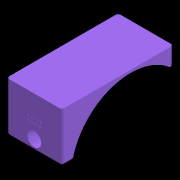
# Autodesk Inventor part: strut_hole
Saved by Autodesk Inventor 2020.2 (Build 242310000, 310)
## iProperties
Created: 2020-04-29
Part Number: strut_hole
Material: PC/ABS Plastic
Document SubType Name: Modeling
Designer: agmlego
Mass: 206.183 g
Surface Area: 707.007 cm^2
Volume: 577.101 cm^3
Density: 0.357273 g/cm^3
Appearance: Violet
Author: agmlego
Autodesk Inventor part; units mm, degrees
ref_plane "YZ Plane" through (0, 0, 0) normal (1, 0, 0) x (0, 1, 0)
ref_plane "XZ Plane" through (0, 0, 0) normal (0, 1, 0) x (-1, 0, 0)
ref_plane "XY Plane" through (0, 0, 0) normal (0, 0, 1) x (1, 0, 0)
sketch "Sketch1" plane through (0, 0, 0) normal (1, 0, 0) x (0, 1, 0)
  arc A0 (76.4375, -78.4587) -> (23.4861, 106.99) centre (0, 0) ccw
  line L0 (114.5375, 126.6449) -> (76.4375, 126.6449)
  line L1 (76.4375, -78.4587) -> (114.5375, -78.4587)
  line L2 (114.5375, -78.4587) -> (114.5375, 126.6449)
  line L3 (114.5375, 0) -> (109.5375, 0) construction
  line L4 (55.1307, 126.6449) -> (28.4861, 126.6449) construction
  line L5 (28.4861, 126.6449) -> (28.4861, 75.8449) construction
  line L6 (28.4861, 75.8449) -> (55.1307, 75.8449) construction
  line L7 (55.1307, 75.8449) -> (55.1307, 126.6449) construction
  line L8 (41.8084, 75.8449) -> (41.8084, 126.6449) construction
  line L9 (76.4375, 126.6449) -> (23.4861, 126.6449)
  line L10 (23.4861, 126.6449) -> (23.4861, 106.99)
  point P0 (41.8084, 101.2449)
  dimension "d0" = 219.075
  dimension "d1" = 38.1
  dimension "d3" = 5
  dimension "d4" = 26.6446
  dimension "d5" = 41.8084
  dimension "d6" = 25.4
  dimension "d7" = 5
  constraints: 22 end point, 4 horizontal, 4 parallel, 4 point on circle, 3 midpoint, 2 perpendicular, 2 point on line, 1 centre point, 1 coincident, 1 collinear, 1 vertical
  measures "d0" diameter of A0
  measures "d1" distance of L0.start L0.end
  measures "d3" distance of L3.start L3.end
  measures "d4" distance of L4.start L4.end
  measures "d5" distance from line of point (0, 0) L8
  measures "d6" distance from line of point (41.808, 101.245) L4
  measures "d7" distance between parallel lines of L5 L10
extrude "Extrusion1" add sketch "Sketch1" along normal blind 101.6
sketch "Sketch3" plane through (0, 23.4861, 126.6449) normal (0, 0, 1) x (1, 0, 0)
  line L0 (0, 18.3223) -> (101.6, 18.3223) construction
  line L1 (101.6, 86.0514) -> (101.6, 0) construction
  point P0 (0, -23.4861)
  point P1 (50.8, 18.3223)
  point P2 (101.6, 52.9514)
  point P3 (50.8, 18.3223)
  dimension "d10" = 41.8084
  constraints: 2 end point, 1 coincident, 1 horizontal, 1 midpoint, 1 point on line
  measures "d10" distance from line of point (0, -23.486) L0
hole "Hole1" at (50.8, 41.8084, 126.6449) direction (0, 0, -1) diameter 25.4 end through all
fillet "Fillet1" radius 5 9 edges at (50.8, 76.4375, -78.4587) (0, 95.4875, -78.4587) (101.6, 95.4875, -78.4587) (0, 69.0118, 126.6449) (50.8, 23.4861, 106.99) (0, 23.4861, 116.8174) (50.8, 23.4861, 126.6449) (101.6, 69.0118, 126.6449) (101.6, 23.4861, 116.8174)
sketch "Sketch4" plane through (5, 28.4861, 126.6449) normal (0, 0, 1) x (1, 0, 0)
  line L0 (32.0406, 47.3735) -> (60.3413, 47.3735) construction
  line L1 (60.3413, 47.3735) -> (60.3413, 37.5666) construction
  line L2 (60.3413, 37.5666) -> (32.0406, 37.5666) construction
  line L3 (32.0406, 37.5666) -> (32.0406, 47.3735) construction
  spline S0 degree 2 poles (35.6936, 46.8807) (35.5562, 46.9611) (35.3046, 47.0363) (35.1516, 47.0363) knots 0 0 0 1 2 2 2
  spline S1 degree 2 poles (35.1516, 47.0363) (35.0426, 47.0363) (34.8352, 46.9922) (34.677, 46.8937) (34.5784, 46.7355) (34.5784, 46.6214) knots 0 0 0 1 2 3 4 4 4
  spline S2 degree 2 poles (34.5784, 46.6214) (34.5784, 46.5098) (34.6977, 46.3439) (34.8922, 46.2142) (35.1438, 46.1027) (35.4057, 45.9808) (35.6573, 45.8355) (35.8518, 45.6358) (35.9711, 45.3713) (35.9711, 45.1897) knots 0 0 0 1 2 3 4 5 6 7 8 8 8
  spline S3 degree 2 poles (35.9711, 45.1897) (35.9711, 45.0419) (35.8907, 44.7903) (35.7481, 44.5906) (35.551, 44.4402) (35.3176, 44.339) (35.0608, 44.2898) (34.9259, 44.2898) knots 0 0 0 1 2 3 4 5 6 6 6
  spline S4 degree 2 poles (34.9259, 44.2898) (34.4565, 44.2976) (34.109, 44.5128) knots 0 0 0 1 1 1
  line L4 (34.109, 44.5128) -> (34.2931, 44.8137)
  spline S5 degree 2 poles (34.2931, 44.8137) (34.332, 44.7877) (34.4643, 44.7229) (34.6251, 44.6606) (34.804, 44.6217) (34.8974, 44.6217) knots 0 0 0 1 2 3 4 4 4
  spline S6 degree 2 poles (34.8974, 44.6217) (35.0219, 44.6217) (35.2605, 44.684) (35.4472, 44.8137) (35.5613, 45.016) (35.5613, 45.1534) knots 0 0 0 1 2 3 4 4 4
  spline S7 degree 2 poles (35.5613, 45.1534) (35.5613, 45.2831) (35.442, 45.4776) (35.2475, 45.6332) (34.996, 45.7577) (34.734, 45.8822) (34.4824, 46.0171) (34.2879, 46.1908) (34.1686, 46.4139) (34.1686, 46.5643) knots 0 0 0 1 2 3 4 5 6 7 8 8 8
  spline S8 degree 2 poles (34.1686, 46.5643) (34.1686, 46.7588) (34.3294, 47.0571) (34.5914, 47.262) (34.9259, 47.3683) (35.0971, 47.3683) knots 0 0 0 1 2 3 4 4 4
  spline S9 degree 2 poles (35.0971, 47.3683) (35.525, 47.3683) (35.8881, 47.1271) knots 0 0 0 1 1 1
  line L5 (35.8881, 47.1271) -> (35.6936, 46.8807)
  line L6 (37.146, 44.3235) -> (37.146, 47.013)
  line L7 (37.146, 47.013) -> (36.3135, 47.013)
  line L8 (36.3135, 47.013) -> (36.3135, 47.3346)
  line L9 (36.3135, 47.3346) -> (38.3909, 47.3346)
  line L10 (38.3909, 47.3346) -> (38.3909, 47.013)
  line L11 (38.3909, 47.013) -> (37.5687, 47.013)
  line L12 (37.5687, 47.013) -> (37.5687, 44.3235)
  line L13 (37.5687, 44.3235) -> (37.146, 44.3235)
  line L14 (39.3661, 45.5554) -> (39.3661, 44.3235)
  line L15 (39.3661, 44.3235) -> (38.9433, 44.3235)
  line L16 (38.9433, 44.3235) -> (38.9433, 46.9118)
  line L17 (38.9433, 46.9118) -> (38.8733, 47.3138)
  spline S10 degree 2 poles (38.8733, 47.3138) (38.9381, 47.3216) (39.1249, 47.3372) (39.3298, 47.3501) (39.5321, 47.3579) (39.6202, 47.3579) knots 0 0 0 1 2 3 4 4 4
  spline S11 degree 2 poles (39.6202, 47.3579) (39.8718, 47.3579) (40.2894, 47.2516) (40.5876, 47.0441) (40.751, 46.7329) (40.751, 46.528) knots 0 0 0 1 2 3 4 4 4
  spline S12 degree 2 poles (40.751, 46.528) (40.751, 46.3179) (40.6213, 45.9963) (40.3827, 45.7707) (40.0559, 45.628) (39.8614, 45.5943) knots 0 0 0 1 2 3 4 4 4
  line L18 (39.8614, 45.5943) -> (40.1467, 45.5139)
  line L19 (40.1467, 45.5139) -> (41.0363, 44.3235)
  line L20 (41.0363, 44.3235) -> (40.5876, 44.3235)
  line L21 (40.5876, 44.3235) -> (39.7006, 45.5165)
  spline S13 degree 2 poles (39.7006, 45.5165) (39.6773, 45.545) (39.6228, 45.5554) (39.6073, 45.5554) knots 0 0 0 1 2 2 2
  line L22 (39.6073, 45.5554) -> (39.3661, 45.5554)
  line L23 (39.3661, 46.624) -> (39.3661, 45.8589)
  line L24 (39.3661, 45.8589) -> (39.6617, 45.8589)
  spline S14 degree 2 poles (39.6617, 45.8589) (39.8459, 45.8589) (40.113, 45.96) (40.2894, 46.1364) (40.3775, 46.3672) (40.3775, 46.4969) knots 0 0 0 1 2 3 4 4 4
  spline S15 degree 2 poles (40.3775, 46.4969) (40.3775, 46.668) (40.2505, 46.8937) (40.0456, 47.0285) (39.794, 47.083) (39.6695, 47.083) knots 0 0 0 1 2 3 4 4 4
  spline S16 degree 2 poles (39.6695, 47.083) (39.628, 47.083) (39.5372, 47.0804) (39.4439, 47.0778) (39.3583, 47.0649) (39.3272, 47.0597) knots 0 0 0 1 2 3 4 4 4
  line L25 (39.3272, 47.0597) -> (39.3661, 46.624)
  line L26 (43.6221, 47.3346) -> (43.6221, 45.3739)
  spline S17 degree 2 poles (43.6221, 45.3739) (43.6221, 45.1015) (43.4561, 44.6944) (43.1708, 44.4246) (42.7766, 44.2898) (42.5457, 44.2898) knots 0 0 0 1 2 3 4 4 4
  spline S18 degree 2 poles (42.5457, 44.2898) (42.302, 44.2898) (41.9233, 44.4609) (41.6665, 44.7722) (41.5317, 45.2079) (41.5317, 45.4724) knots 0 0 0 1 2 3 4 4 4
  line L27 (41.5317, 45.4724) -> (41.5317, 46.9118)
  line L28 (41.5317, 46.9118) -> (41.472, 47.3346)
  line L29 (41.472, 47.3346) -> (41.944, 47.3735)
  line L30 (41.944, 47.3735) -> (41.944, 45.4361)
  spline S19 degree 2 poles (41.944, 45.4361) (41.944, 45.2468) (42.0452, 44.9459) (42.2164, 44.741) (42.4394, 44.6321) (42.5665, 44.6321) knots 0 0 0 1 2 3 4 4 4
  spline S20 degree 2 poles (42.5665, 44.6321) (42.7143, 44.6321) (42.9529, 44.7203) (43.1189, 44.8967) (43.2097, 45.1586) (43.2097, 45.3376) knots 0 0 0 1 2 3 4 4 4
  line L31 (43.2097, 45.3376) -> (43.2097, 47.3346)
  line L32 (43.2097, 47.3346) -> (43.6221, 47.3346)
  line L33 (44.9759, 44.3235) -> (44.9759, 47.013)
  line L34 (44.9759, 47.013) -> (44.1434, 47.013)
  line L35 (44.1434, 47.013) -> (44.1434, 47.3346)
  line L36 (44.1434, 47.3346) -> (46.2208, 47.3346)
  line L37 (46.2208, 47.3346) -> (46.2208, 47.013)
  line L38 (46.2208, 47.013) -> (45.3986, 47.013)
  line L39 (45.3986, 47.013) -> (45.3986, 44.3235)
  line L40 (45.3986, 44.3235) -> (44.9759, 44.3235)
  line L41 (49.8362, 44.3235) -> (49.8362, 45.7785)
  line L42 (49.8362, 45.7785) -> (48.5705, 45.7785)
  line L43 (48.5705, 45.7785) -> (48.5705, 44.3235)
  line L44 (48.5705, 44.3235) -> (48.1582, 44.3235)
  line L45 (48.1582, 44.3235) -> (48.1582, 46.9118)
  line L46 (48.1582, 46.9118) -> (48.1011, 47.3346)
  line L47 (48.1011, 47.3346) -> (48.5705, 47.3735)
  line L48 (48.5705, 47.3735) -> (48.5705, 46.1001)
  line L49 (48.5705, 46.1001) -> (49.8362, 46.1001)
  line L50 (49.8362, 46.1001) -> (49.8362, 47.3372)
  line L51 (49.8362, 47.3372) -> (50.2486, 47.3735)
  line L52 (50.2486, 47.3735) -> (50.2486, 44.3235)
  line L53 (50.2486, 44.3235) -> (49.8362, 44.3235)
  spline S21 degree 2 poles (52.2145, 44.2898) (51.898, 44.2898) (51.3949, 44.5232) (51.0448, 44.933) (50.858, 45.4984) (50.858, 45.8303) knots 0 0 0 1 2 3 4 4 4
  spline S22 degree 2 poles (50.858, 45.8303) (50.858, 46.1597) (51.0396, 46.7251) (51.3845, 47.1349) (51.8903, 47.3683) (52.2145, 47.3683) knots 0 0 0 1 2 3 4 4 4
  spline S23 degree 2 poles (52.2145, 47.3683) (52.5283, 47.3683) (53.034, 47.1349) (53.3841, 46.7251) (53.5709, 46.1597) (53.5709, 45.8303) knots 0 0 0 1 2 3 4 4 4
  spline S24 degree 2 poles (53.5709, 45.8303) (53.5709, 45.4984) (53.3893, 44.933) (53.0444, 44.5232) (52.5386, 44.2898) (52.2145, 44.2898) knots 0 0 0 1 2 3 4 4 4
  spline S25 degree 2 poles (53.1533, 45.7681) (53.1533, 45.9263) (53.1092, 46.2375) (53.0133, 46.5176) (52.8602, 46.7562) (52.6502, 46.9274) (52.3753, 47.026) (52.2015, 47.026) knots 0 0 0 1 2 3 4 5 6 6 6
  spline S26 degree 2 poles (52.2015, 47.026) (51.9551, 47.026) (51.605, 46.8366) (51.3793, 46.5176) (51.2756, 46.113) (51.2756, 45.9004) knots 0 0 0 1 2 3 4 4 4
  spline S27 degree 2 poles (51.2756, 45.9004) (51.2756, 45.737) (51.3223, 45.4231) (51.4182, 45.1404) (51.5687, 44.9018) (51.7787, 44.7307) (52.0537, 44.6321) (52.2274, 44.6321) knots 0 0 0 1 2 3 4 5 6 6 6
  spline S28 degree 2 poles (52.2274, 44.6321) (52.3882, 44.6321) (52.6528, 44.7229) (52.8602, 44.8785) (53.0081, 45.0964) (53.1066, 45.3453) (53.1533, 45.6254) (53.1533, 45.7681) knots 0 0 0 1 2 3 4 5 6 6 6
  line L54 (54.6031, 44.6451) -> (55.9076, 44.6451)
  line L55 (55.9076, 44.6451) -> (55.8687, 44.3235)
  line L56 (55.8687, 44.3235) -> (54.1622, 44.3235)
  line L57 (54.1622, 44.3235) -> (54.2011, 44.7255)
  line L58 (54.2011, 44.7255) -> (54.2011, 46.9118)
  line L59 (54.2011, 46.9118) -> (54.1415, 47.3346)
  line L60 (54.1415, 47.3346) -> (54.6238, 47.3735)
  line L61 (54.6238, 47.3735) -> (54.6238, 45.0056)
  line L62 (54.6238, 45.0056) -> (54.6031, 44.6451)
  line L63 (58.1251, 44.6451) -> (58.0862, 44.3235)
  line L64 (58.0862, 44.3235) -> (56.3771, 44.3235)
  line L65 (56.3771, 44.3235) -> (56.4082, 44.7255)
  line L66 (56.4082, 44.7255) -> (56.4082, 46.9118)
  line L67 (56.4082, 46.9118) -> (56.3486, 47.3346)
  line L68 (56.3486, 47.3346) -> (58.0551, 47.3346)
  line L69 (58.0551, 47.3346) -> (58.0551, 47.013)
  line L70 (58.0551, 47.013) -> (56.7895, 47.013)
  line L71 (56.7895, 47.013) -> (56.8309, 46.6317)
  line L72 (56.8309, 46.6317) -> (56.8309, 46.1001)
  line L73 (56.8309, 46.1001) -> (57.915, 46.1001)
  line L74 (57.915, 46.1001) -> (57.915, 45.8122)
  line L75 (57.915, 45.8122) -> (56.8309, 45.8122)
  line L76 (56.8309, 45.8122) -> (56.8309, 45.0082)
  line L77 (56.8309, 45.0082) -> (56.8102, 44.6451)
  line L78 (56.8102, 44.6451) -> (58.1251, 44.6451)
  line L79 (32.7409, 37.6003) -> (32.7409, 37.9219)
  line L80 (32.7409, 37.9219) -> (33.2336, 37.9219)
  line L81 (33.2336, 37.9219) -> (33.2336, 39.8593)
  line L82 (33.2336, 39.8593) -> (33.3504, 40.3158)
  line L83 (33.3504, 40.3158) -> (33.078, 39.9423)
  line L84 (33.078, 39.9423) -> (32.6527, 39.5662)
  line L85 (32.6527, 39.5662) -> (32.4348, 39.8074)
  line L86 (32.4348, 39.8074) -> (33.3555, 40.6503)
  line L87 (33.3555, 40.6503) -> (33.6564, 40.6114)
  line L88 (33.6564, 40.6114) -> (33.6564, 37.9219)
  line L89 (33.6564, 37.9219) -> (34.1492, 37.9219)
  line L90 (34.1492, 37.9219) -> (34.1492, 37.6003)
  line L91 (34.1492, 37.6003) -> (32.7409, 37.6003)
  line L92 (35.905, 40.6114) -> (35.905, 40.4117)
  spline S29 degree 2 poles (35.905, 40.4117) (35.905, 40.3339) (35.8765, 40.1109) (35.8609, 40.0019) knots 0 0 0 1 2 2 2
  spline S30 degree 2 poles (35.8609, 40.0019) (35.8402, 39.8775) (35.8168, 39.7426) knots 0 0 0 1 1 1
  line L93 (35.8168, 39.7426) -> (35.643, 39.7426)
  spline S31 degree 2 poles (35.643, 39.7426) (35.6197, 39.8775) (35.599, 40.0019) knots 0 0 0 1 1 1
  spline S32 degree 2 poles (35.599, 40.0019) (35.5834, 40.1109) (35.5549, 40.3339) (35.5549, 40.4117) knots 0 0 0 1 2 2 2
  line L94 (35.5549, 40.4117) -> (35.5549, 40.6114)
  line L95 (35.5549, 40.6114) -> (35.905, 40.6114)
  line L96 (35.3007, 40.6114) -> (35.3007, 40.4117)
  spline S33 degree 2 poles (35.3007, 40.4117) (35.3007, 40.3339) (35.2722, 40.1109) (35.2566, 40.0019) knots 0 0 0 1 2 2 2
  spline S34 degree 2 poles (35.2566, 40.0019) (35.2359, 39.8775) (35.2125, 39.7426) knots 0 0 0 1 1 1
  line L97 (35.2125, 39.7426) -> (35.0387, 39.7426)
  spline S35 degree 2 poles (35.0387, 39.7426) (35.0154, 39.8775) (34.9947, 40.0019) knots 0 0 0 1 1 1
  spline S36 degree 2 poles (34.9947, 40.0019) (34.9791, 40.1109) (34.9506, 40.3339) (34.9506, 40.4117) knots 0 0 0 1 2 2 2
  line L98 (34.9506, 40.4117) -> (34.9506, 40.6114)
  line L99 (34.9506, 40.6114) -> (35.3007, 40.6114)
  line L100 (38.4648, 37.6003) -> (38.0421, 37.6003)
  line L101 (38.0421, 37.6003) -> (38.0421, 40.1887)
  line L102 (38.0421, 40.1887) -> (37.9824, 40.6114)
  line L103 (37.9824, 40.6114) -> (39.759, 40.6114)
  line L104 (39.759, 40.6114) -> (39.7201, 40.2898)
  line L105 (39.7201, 40.2898) -> (38.4259, 40.2898)
  line L106 (38.4259, 40.2898) -> (38.4648, 39.9086)
  line L107 (38.4648, 39.9086) -> (38.4648, 39.3769)
  line L108 (38.4648, 39.3769) -> (39.5489, 39.3769)
  line L109 (39.5489, 39.3769) -> (39.5489, 39.089)
  line L110 (39.5489, 39.089) -> (38.4648, 39.089)
  line L111 (38.4648, 39.089) -> (38.4648, 37.6003)
  spline S37 degree 2 poles (41.0687, 37.5666) (40.8457, 37.5666) (40.48, 37.7404) (40.2155, 38.049) (40.0676, 38.4692) (40.0676, 38.7104) knots 0 0 0 1 2 3 4 4 4
  spline S38 degree 2 poles (40.0676, 38.7104) (40.0676, 38.9542) (40.2077, 39.3691) (40.4696, 39.6726) (40.8405, 39.8437) (41.0687, 39.8437) knots 0 0 0 1 2 3 4 4 4
  spline S39 degree 2 poles (41.0687, 39.8437) (41.2918, 39.8437) (41.6626, 39.6726) (41.9272, 39.3691) (42.075, 38.9542) (42.075, 38.7104) knots 0 0 0 1 2 3 4 4 4
  spline S40 degree 2 poles (42.075, 38.7104) (42.075, 38.4692) (41.9324, 38.049) (41.6704, 37.7404) (41.297, 37.5666) (41.0687, 37.5666) knots 0 0 0 1 2 3 4 4 4
  spline S41 degree 2 poles (41.6938, 38.6559) (41.6938, 38.8193) (41.6237, 39.1331) (41.4707, 39.3795) (41.2295, 39.5325) (41.0609, 39.5325) knots 0 0 0 1 2 3 4 4 4
  spline S42 degree 2 poles (41.0609, 39.5325) (40.9001, 39.5325) (40.6667, 39.4002) (40.5189, 39.1798) (40.4489, 38.8971) (40.4489, 38.7493) knots 0 0 0 1 2 3 4 4 4
  spline S43 degree 2 poles (40.4489, 38.7493) (40.4489, 38.5859) (40.5189, 38.2747) (40.6693, 38.0283) (40.9079, 37.8778) (41.0765, 37.8778) knots 0 0 0 1 2 3 4 4 4
  spline S44 degree 2 poles (41.0765, 37.8778) (41.2347, 37.8778) (41.4681, 38.0101) (41.6211, 38.2306) (41.6938, 38.5107) (41.6938, 38.6559) knots 0 0 0 1 2 3 4 4 4
  spline S45 degree 2 poles (43.626, 39.504) (43.5456, 39.504) (43.3873, 39.4391) (43.2421, 39.3302) (43.115, 39.1876) (43.0606, 39.1072) knots 0 0 0 1 2 3 4 4 4
  line L112 (43.0606, 39.1072) -> (43.0606, 37.6003)
  line L113 (43.0606, 37.6003) -> (42.6793, 37.6003)
  line L114 (42.6793, 37.6003) -> (42.6793, 39.81)
  line L115 (42.6793, 39.81) -> (43.0606, 39.8489)
  line L116 (43.0606, 39.8489) -> (43.0606, 39.3977)
  line L117 (43.0606, 39.3977) -> (43.2603, 39.7504)
  spline S46 degree 2 poles (43.2603, 39.7504) (43.2862, 39.7659) (43.3666, 39.7997) (43.4652, 39.8256) (43.5793, 39.8437) (43.6415, 39.8437) knots 0 0 0 1 2 3 4 4 4
  spline S47 degree 2 poles (43.6415, 39.8437) (43.7323, 39.8437) (43.8542, 39.8126) (43.8827, 39.7971) knots 0 0 0 1 2 2 2
  line L118 (43.8827, 39.7971) -> (43.8646, 39.4651)
  spline S48 degree 2 poles (43.8646, 39.4651) (43.8334, 39.4729) (43.7141, 39.504) (43.626, 39.504) knots 0 0 0 1 2 2 2
  spline S49 degree 2 poles (45.2106, 39.4469) (45.1743, 39.4651) (45.0731, 39.5014) (44.9642, 39.5299) (44.8553, 39.5455) (44.806, 39.5455) knots 0 0 0 1 2 3 4 4 4
  spline S50 degree 2 poles (44.806, 39.5455) (44.5933, 39.5455) (44.417, 39.4184) (44.417, 39.2913) knots 0 0 0 1 2 2 2
  spline S51 degree 2 poles (44.417, 39.2913) (44.417, 39.2083) (44.5337, 39.0968) (44.7178, 39.0086) (44.9435, 38.9308) (45.0524, 38.8764) knots 0 0 0 1 2 3 4 4 4
  spline S52 degree 2 poles (45.0524, 38.8764) (45.1302, 38.8374) (45.291, 38.7337) (45.4181, 38.5937) (45.4985, 38.4173) (45.4985, 38.3058) knots 0 0 0 1 2 3 4 4 4
  spline S53 degree 2 poles (45.4985, 38.3058) (45.4985, 38.1035) (45.361, 37.8208) (45.1276, 37.647) (44.8138, 37.5666) (44.6348, 37.5666) knots 0 0 0 1 2 3 4 4 4
  spline S54 degree 2 poles (44.6348, 37.5666) (44.5648, 37.5666) (44.3936, 37.5926) (44.2199, 37.6392) (44.0643, 37.7041) (44.0124, 37.7404) knots 0 0 0 1 2 3 4 4 4
  line L119 (44.0124, 37.7404) -> (44.1447, 38.0049)
  spline S55 degree 2 poles (44.1447, 38.0049) (44.1939, 37.9816) (44.3262, 37.9375) (44.4663, 37.9064) (44.6037, 37.8882) (44.6582, 37.8882) knots 0 0 0 1 2 3 4 4 4
  spline S56 degree 2 poles (44.6582, 37.8882) (44.7515, 37.8882) (44.9227, 37.9271) (45.0524, 38.0101) (45.1302, 38.145) (45.1302, 38.2435) knots 0 0 0 1 2 3 4 4 4
  spline S57 degree 2 poles (45.1302, 38.2435) (45.1302, 38.3187) (45.068, 38.4303) (44.9616, 38.5158) (44.8216, 38.5885) (44.6634, 38.6559) (44.5, 38.7259) (44.4248, 38.7674) knots 0 0 0 1 2 3 4 5 6 6 6
  spline S58 degree 2 poles (44.4248, 38.7674) (44.3547, 38.8089) (44.2251, 38.9049) (44.1239, 39.0242) (44.0643, 39.1746) (44.0643, 39.2706) knots 0 0 0 1 2 3 4 4 4
  spline S59 degree 2 poles (44.0643, 39.2706) (44.0643, 39.4236) (44.1732, 39.644) (44.3703, 39.7789) (44.6452, 39.8437) (44.8112, 39.8437) knots 0 0 0 1 2 3 4 4 4
  spline S60 degree 2 poles (44.8112, 39.8437) (44.889, 39.8437) (45.0368, 39.8204) (45.1743, 39.7815) (45.2858, 39.7296) (45.3247, 39.7037) knots 0 0 0 1 2 3 4 4 4
  line L120 (45.3247, 39.7037) -> (45.2106, 39.4469)
  spline S61 degree 2 poles (46.4737, 38.3551) (46.4737, 38.2228) (46.5048, 38.0438) (46.5618, 37.9349) (46.6474, 37.8882) (46.7045, 37.8882) knots 0 0 0 1 2 3 4 4 4
  spline S62 degree 2 poles (46.7045, 37.8882) (46.7486, 37.8882) (46.8212, 37.8986) (46.8471, 37.9064) knots 0 0 0 1 2 2 2
  spline S63 degree 2 poles (46.8471, 37.9064) (46.8782, 37.9141) (46.9016, 37.9245) knots 0 0 0 1 1 1
  line L121 (46.9016, 37.9245) -> (47.039, 37.6807)
  spline S64 degree 2 poles (47.039, 37.6807) (47.0235, 37.6652) (46.9535, 37.6263) (46.8575, 37.59) (46.7356, 37.5666) (46.6656, 37.5666) knots 0 0 0 1 2 3 4 4 4
  spline S65 degree 2 poles (46.6656, 37.5666) (46.484, 37.5666) (46.2584, 37.6989) (46.1339, 37.9271) (46.0924, 38.2306) (46.0924, 38.4017) knots 0 0 0 1 2 3 4 4 4
  line L122 (46.0924, 38.4017) -> (46.0924, 39.4858)
  line L123 (46.0924, 39.4858) -> (45.7916, 39.4858)
  line L124 (45.7916, 39.4858) -> (45.7916, 39.8074)
  line L125 (45.7916, 39.8074) -> (46.0924, 39.8074)
  line L126 (46.0924, 39.8074) -> (46.0924, 40.2276)
  line L127 (46.0924, 40.2276) -> (46.4633, 40.4506)
  line L128 (46.4633, 40.4506) -> (46.4633, 39.8074)
  line L129 (46.4633, 39.8074) -> (47.1454, 39.8074)
  line L130 (47.1454, 39.8074) -> (47.1065, 39.4858)
  line L131 (47.1065, 39.4858) -> (46.4737, 39.4858)
  line L132 (46.4737, 39.4858) -> (46.4737, 38.3551)
  line L133 (48.0791, 37.6003) -> (47.6978, 37.6003)
  line L134 (47.6978, 37.6003) -> (47.6978, 39.81)
  line L135 (47.6978, 39.81) -> (48.0791, 39.8489)
  line L136 (48.0791, 39.8489) -> (48.0791, 39.4806)
  line L137 (48.0791, 39.4806) -> (48.201, 39.6959)
  spline S66 degree 2 poles (48.201, 39.6959) (48.2373, 39.7218) (48.3488, 39.7737) (48.4888, 39.8152) (48.6496, 39.8437) (48.73, 39.8437) knots 0 0 0 1 2 3 4 4 4
  spline S67 degree 2 poles (48.73, 39.8437) (48.8908, 39.8437) (49.1087, 39.7426) (49.2461, 39.5481) (49.3032, 39.2758) (49.3032, 39.1072) knots 0 0 0 1 2 3 4 4 4
  line L138 (49.3032, 39.1072) -> (49.3032, 37.6003)
  line L139 (49.3032, 37.6003) -> (48.922, 37.6003)
  line L140 (48.922, 37.6003) -> (48.922, 39.1072)
  spline S68 degree 2 poles (48.922, 39.1072) (48.922, 39.2161) (48.8908, 39.3717) (48.8182, 39.4729) (48.6937, 39.5221) (48.6004, 39.5221) knots 0 0 0 1 2 3 4 4 4
  spline S69 degree 2 poles (48.6004, 39.5221) (48.5329, 39.5221) (48.3929, 39.4806) (48.258, 39.4132) (48.1309, 39.3328) (48.0791, 39.2965) knots 0 0 0 1 2 3 4 4 4
  line L141 (48.0791, 39.2965) -> (48.0791, 37.6003)
  spline S70 degree 2 poles (51.6426, 37.8597) (51.5803, 37.7948) (51.4325, 37.6885) (51.251, 37.6081) (51.0331, 37.5666) (50.8982, 37.5666) knots 0 0 0 1 2 3 4 4 4
  spline S71 degree 2 poles (50.8982, 37.5666) (50.6311, 37.5666) (50.255, 37.7559) (50.0164, 38.0724) (49.9049, 38.4821) (49.9049, 38.7052) knots 0 0 0 1 2 3 4 4 4
  spline S72 degree 2 poles (49.9049, 38.7052) (49.9049, 38.8478) (49.9568, 39.1279) (50.0605, 39.3795) (50.2187, 39.5974) (50.4262, 39.753) (50.6907, 39.8437) (50.849, 39.8437) knots 0 0 0 1 2 3 4 5 6 6 6
  spline S73 degree 2 poles (50.849, 39.8437) (51.0642, 39.8437) (51.3832, 39.7037) (51.5907, 39.4495) (51.6919, 39.0968) (51.6919, 38.8815) knots 0 0 0 1 2 3 4 4 4
  spline S74 degree 2 poles (51.6919, 38.8815) (51.6919, 38.8193) (51.6841, 38.6715) (51.6763, 38.604) knots 0 0 0 1 2 2 2
  line L142 (51.6763, 38.604) -> (50.2862, 38.604)
  spline S75 degree 2 poles (50.2862, 38.604) (50.2862, 38.4536) (50.3691, 38.1943) (50.517, 37.9997) (50.7271, 37.8882) (50.8593, 37.8882) knots 0 0 0 1 2 3 4 4 4
  spline S76 degree 2 poles (50.8593, 37.8882) (50.9864, 37.8882) (51.1783, 37.9271) (51.3132, 37.9816) (51.4014, 38.036) (51.4247, 38.0516) knots 0 0 0 1 2 3 4 4 4
  line L143 (51.4247, 38.0516) -> (51.6426, 37.8597)
  spline S77 degree 2 poles (51.3106, 38.9049) (51.3132, 38.9282) (51.3158, 38.9723) (51.3158, 38.9931) knots 0 0 0 1 2 2 2
  spline S78 degree 2 poles (51.3158, 38.9931) (51.3158, 39.1072) (51.2613, 39.3017) (51.155, 39.4443) (50.9916, 39.5247) (50.8775, 39.5247) knots 0 0 0 1 2 3 4 4 4
  spline S79 degree 2 poles (50.8775, 39.5247) (50.7452, 39.5247) (50.5533, 39.4391) (50.4236, 39.3043) (50.3432, 39.1435) (50.3251, 39.0709) knots 0 0 0 1 2 3 4 4 4
  line L144 (50.3251, 39.0709) -> (50.2187, 38.8504)
  line L145 (50.2187, 38.8504) -> (50.5766, 38.9049)
  line L146 (50.5766, 38.9049) -> (51.3106, 38.9049)
  spline S80 degree 2 poles (53.2609, 39.504) (53.1805, 39.504) (53.0223, 39.4391) (52.8771, 39.3302) (52.75, 39.1876) (52.6956, 39.1072) knots 0 0 0 1 2 3 4 4 4
  line L147 (52.6956, 39.1072) -> (52.6956, 37.6003)
  line L148 (52.6956, 37.6003) -> (52.3143, 37.6003)
  line L149 (52.3143, 37.6003) -> (52.3143, 39.81)
  line L150 (52.3143, 39.81) -> (52.6956, 39.8489)
  line L151 (52.6956, 39.8489) -> (52.6956, 39.3977)
  line L152 (52.6956, 39.3977) -> (52.8953, 39.7504)
  spline S81 degree 2 poles (52.8953, 39.7504) (52.9212, 39.7659) (53.0016, 39.7997) (53.1001, 39.8256) (53.2143, 39.8437) (53.2765, 39.8437) knots 0 0 0 1 2 3 4 4 4
  spline S82 degree 2 poles (53.2765, 39.8437) (53.3673, 39.8437) (53.4892, 39.8126) (53.5177, 39.7971) knots 0 0 0 1 2 2 2
  line L153 (53.5177, 39.7971) -> (53.4995, 39.4651)
  spline S83 degree 2 poles (53.4995, 39.4651) (53.4684, 39.4729) (53.3491, 39.504) (53.2609, 39.504) knots 0 0 0 1 2 2 2
  line L154 (55.3047, 37.6003) -> (55.3047, 40.1913)
  line L155 (55.3047, 40.1913) -> (55.245, 40.5933)
  spline S84 degree 2 poles (55.245, 40.5933) (55.3047, 40.6011) (55.4629, 40.6166) (55.6314, 40.627) (55.7974, 40.6322) (55.8623, 40.6322) knots 0 0 0 1 2 3 4 4 4
  spline S85 degree 2 poles (55.8623, 40.6322) (56.0827, 40.6322) (56.5003, 40.5751) (56.8219, 40.4221) (57.0138, 40.155) (57.0138, 39.9475) knots 0 0 0 1 2 3 4 4 4
  spline S86 degree 2 poles (57.0138, 39.9475) (57.0138, 39.7296) (56.8037, 39.4106) (56.6299, 39.3276) knots 0 0 0 1 2 2 2
  line L156 (56.6299, 39.3276) -> (56.3213, 39.2394)
  line L157 (56.3213, 39.2394) -> (56.617, 39.2109)
  spline S87 degree 2 poles (56.617, 39.2109) (56.7389, 39.1746) (56.9567, 39.0605) (57.1227, 38.8945) (57.2161, 38.6715) (57.2161, 38.5236) knots 0 0 0 1 2 3 4 4 4
  spline S88 degree 2 poles (57.2161, 38.5236) (57.2161, 38.3525) (57.1227, 38.0853) (56.9671, 37.8804) (56.7544, 37.7326) (56.5106, 37.6418) (56.2513, 37.6003) (56.1268, 37.6003) knots 0 0 0 1 2 3 4 5 6 6 6
  line L158 (56.1268, 37.6003) -> (55.3047, 37.6003)
  line L159 (55.7274, 37.9219) -> (56.0075, 37.9219)
  spline S89 degree 2 poles (56.0075, 37.9219) (56.2072, 37.9219) (56.5081, 37.979) (56.7129, 38.1139) (56.8141, 38.3369) (56.8141, 38.5029) knots 0 0 0 1 2 3 4 4 4
  spline S90 degree 2 poles (56.8141, 38.5029) (56.8141, 38.6533) (56.7103, 38.866) (56.5184, 39.0034) (56.2513, 39.0657) (56.0879, 39.0657) knots 0 0 0 1 2 3 4 4 4
  line L160 (56.0879, 39.0657) -> (55.7274, 39.0657)
  line L161 (55.7274, 39.0657) -> (55.7274, 37.9219)
  line L162 (55.7274, 39.9034) -> (55.7274, 39.3769)
  line L163 (55.7274, 39.3769) -> (55.9478, 39.3769)
  spline S91 degree 2 poles (55.9478, 39.3769) (56.0775, 39.3769) (56.3239, 39.434) (56.5132, 39.561) (56.6299, 39.7633) (56.6299, 39.906) knots 0 0 0 1 2 3 4 4 4
  spline S92 degree 2 poles (56.6299, 39.906) (56.6299, 40.0383) (56.5184, 40.2146) (56.3343, 40.321) (56.1061, 40.3624) (55.9919, 40.3624) knots 0 0 0 1 2 3 4 4 4
  spline S93 degree 2 poles (55.9919, 40.3624) (55.9582, 40.3624) (55.8778, 40.3573) (55.7948, 40.3495) (55.717, 40.3365) (55.6885, 40.3313) knots 0 0 0 1 2 3 4 4 4
  line L164 (55.6885, 40.3313) -> (55.7274, 39.9034)
  line L165 (58.3157, 37.6003) -> (57.9345, 37.6003)
  line L166 (57.9345, 37.6003) -> (57.9345, 39.7193)
  line L167 (57.9345, 39.7193) -> (58.3157, 39.7607)
  line L168 (58.3157, 39.7607) -> (58.3157, 37.6003)
  line L169 (57.9215, 40.6114) -> (58.3287, 40.6114)
  line L170 (58.3287, 40.6114) -> (58.3287, 40.2094)
  line L171 (58.3287, 40.2094) -> (57.9215, 40.2094)
  line L172 (57.9215, 40.2094) -> (57.9215, 40.6114)
  spline S94 degree 2 poles (59.5191, 38.3551) (59.5191, 38.2228) (59.5503, 38.0438) (59.6073, 37.9349) (59.6929, 37.8882) (59.75, 37.8882) knots 0 0 0 1 2 3 4 4 4
  spline S95 degree 2 poles (59.75, 37.8882) (59.7941, 37.8882) (59.8667, 37.8986) (59.8926, 37.9064) knots 0 0 0 1 2 2 2
  spline S96 degree 2 poles (59.8926, 37.9064) (59.9237, 37.9141) (59.9471, 37.9245) knots 0 0 0 1 1 1
  line L173 (59.9471, 37.9245) -> (60.0845, 37.6807)
  spline S97 degree 2 poles (60.0845, 37.6807) (60.069, 37.6652) (59.999, 37.6263) (59.903, 37.59) (59.7811, 37.5666) (59.7111, 37.5666) knots 0 0 0 1 2 3 4 4 4
  spline S98 degree 2 poles (59.7111, 37.5666) (59.5295, 37.5666) (59.3039, 37.6989) (59.1794, 37.9271) (59.1379, 38.2306) (59.1379, 38.4017) knots 0 0 0 1 2 3 4 4 4
  line L174 (59.1379, 38.4017) -> (59.1379, 39.4858)
  line L175 (59.1379, 39.4858) -> (58.837, 39.4858)
  line L176 (58.837, 39.4858) -> (58.837, 39.8074)
  line L177 (58.837, 39.8074) -> (59.1379, 39.8074)
  line L178 (59.1379, 39.8074) -> (59.1379, 40.2276)
  line L179 (59.1379, 40.2276) -> (59.5088, 40.4506)
  line L180 (59.5088, 40.4506) -> (59.5088, 39.8074)
  line L181 (59.5088, 39.8074) -> (60.1909, 39.8074)
  line L182 (60.1909, 39.8074) -> (60.152, 39.4858)
  line L183 (60.152, 39.4858) -> (59.5191, 39.4858)
  line L184 (59.5191, 39.4858) -> (59.5191, 38.3551)
  point P0 (-5, -28.4861)
  constraints: 2 other
emboss "Emboss1" sketch "Sketch4" operation cut depth 1 direction (0, 0, -1)
equation "\"d0\" = hull_od"
equation "\"hull_od\" = 219.075"
equation "\"hull_id\" = 201.7268"
equation "\"hull_wall\" = 8.6741"
equation "\"hull_length\" = 609.6"
equation "\"hull_spacing\" = 390.525"
equation "\"impeller_od\" = 76.2"
equation "\"impeller_clearance\" = 0.5"
equation "\"impeller_shaft_id\" = 3.175"
equation "\"impeller_shaft_od\" = 5.715"
equation "\"impeller_shaft_support\" = 3.175"
equation "\"impeller_intake_od\" = 19.05"
equation "\"impeller_vane_thick\" = 2"
equation "\"impeller_vane_inner_rad\" = 3.175"
equation "\"impeller_vane_outer_rad\" = 0.37206"
equation "\"magnet_od\" = 5.95"
equation "\"magnet_clearance\" = 0.25"
equation "\"magnet_rad\" = 0.25"
equation "\"magnet_circle_offset\" = 3.175"
equation "\"motor_shaft_od\" = 12.7"
equation "\"motor_shaft_length\" = 31.75"
equation "\"motor_shaft_key\" = 3.048"
equation "\"slab_thick\" = 34.671"
body "Solid1"
